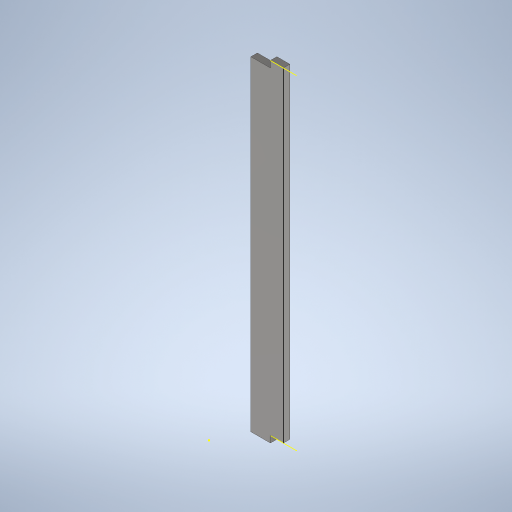
# Autodesk Inventor part: Part2
Saved by Autodesk Inventor 2024 (Build 280153000, 153)
## iProperties
Created: 2023-10-19
Part Number: Part2
Material: Steel, Carbon
Document SubType Name: Modeling
Designer: liuyu
Density: 7.85 g/cm^3
Appearance: Semi-Polished
Author: liuyu
Autodesk Inventor part; units mm, degrees
ref_plane "YZ Plane" through (0, 0, 0) normal (1, 0, 0) x (0, 1, 0)
ref_plane "XZ Plane" through (0, 0, 0) normal (0, 1, 0) x (-1, 0, 0)
ref_plane "XY Plane" through (0, 0, 0) normal (0, 0, 1) x (1, 0, 0)
sketch "Sketch1" plane through (0, 0, 0) normal (0, 0, 1) x (1, 0, 0)
  line L0 (32.1184, 271.7487) -> (82.1184, 271.7487)
  line L1 (82.1184, 271.7487) -> (82.1184, 21.7487)
  line L2 (82.1184, 21.7487) -> (32.1184, 21.7487)
  line L3 (32.1184, 21.7487) -> (32.1184, 271.7487)
  point P0 (0, 0)
  dimension "d0" = 50
  dimension "d1" = 250
  constraints: 8 end point, 2 parallel, 1 horizontal, 1 perpendicular
  measures "d0" distance of L1.end L2.end
  measures "d1" distance of L0.end L1.end
extrude "Extrusion1" add sketch "Sketch1" along normal blind 5
sketch "Sketch2" plane through (0, 0, 5) normal (0, 0, 1) x (1, 0, 0)
  line L0 (82.1184, 271.7487) -> (32.1184, 271.7487) projected
  line L1 (57.1184, 271.7487) -> (47.1184, 271.7487)
  line L2 (47.1184, 271.7487) -> (47.1184, 276.7487)
  line L3 (47.1184, 276.7487) -> (67.1184, 276.7487)
  line L4 (67.1184, 276.7487) -> (67.1184, 271.7487)
  line L5 (32.1184, 21.7487) -> (82.1184, 21.7487) projected
  line L6 (32.1184, 21.7487) -> (32.1184, 16.7487)
  line L7 (32.1184, 16.7487) -> (47.1184, 16.7487)
  line L8 (47.1184, 16.7487) -> (47.1184, 21.7487)
  line L9 (82.1184, 21.7487) -> (82.1184, 16.7487)
  line L10 (82.1184, 16.7487) -> (67.1184, 16.7487)
  line L11 (67.1184, 16.7487) -> (67.1184, 21.7487)
  point P0 (0, 0)
  dimension "d4" = 10
  dimension "d5" = 5
  dimension "d6" = 20
  dimension "d7" = 5
  dimension "d8" = 15
  dimension "d9" = 5
  dimension "d10" = 15
  constraints: 20 end point, 6 point on line, 5 perpendicular, 1 horizontal, 1 midpoint, 1 vertical
  measures "d4" distance of L1.start L1.end
  measures "d5" distance of L1.end L2.end
  measures "d6" distance of L2.end L3.end
  measures "d7" distance of L5.start L6.end
  measures "d8" distance of L6.end L7.end
  measures "d9" distance of L5.end L9.end
  measures "d10" distance of L9.end L10.end
extrude "Extrusion2" add sketch "Sketch2" against normal blind 5 contours L0 L2 L3 L4
sketch "Sketch3" plane through (0, 0, 5) normal (0, 0, 1) x (1, 0, 0)
  line L0 (32.1184, 21.7487) -> (82.1184, 21.7487) projected
  line L1 (32.1184, 21.7487) -> (32.1184, 16.7487)
  line L2 (32.1184, 16.7487) -> (47.1184, 16.7487)
  line L3 (47.1184, 16.7487) -> (47.1184, 21.7487)
  line L4 (82.1184, 21.7487) -> (82.1184, 16.7487)
  line L5 (82.1184, 16.7487) -> (67.1184, 16.7487)
  line L6 (67.1184, 16.7487) -> (67.1184, 21.7487)
  point P0 (0, 0)
  dimension "d13" = 5
  dimension "d14" = 15
  dimension "d15" = 5
  dimension "d16" = 15
  constraints: 12 end point, 4 perpendicular, 2 point on line, 2 vertical
  measures "d13" distance of L0.start L1.end
  measures "d14" distance of L1.end L2.end
  measures "d15" distance of L0.end L4.end
  measures "d16" distance of L4.end L5.end
extrude "Extrusion3" add sketch "Sketch3" against normal blind 5
sketch "Sketch4" plane through (0, 0, 5) normal (0, 0, 1) x (1, 0, 0)
  line L0 (47.1184, 21.7487) -> (67.1184, 21.7487) projected
  line L1 (57.1184, 21.7487) -> (57.1184, 26.7487)
  line L2 (57.1184, 26.7487) -> (47.1184, 26.7487)
  line L3 (47.1184, 26.7487) -> (47.1184, 21.7487)
  line L4 (47.1184, 21.7487) -> (67.1184, 21.7487)
  line L5 (67.1184, 21.7487) -> (67.1184, 26.7487)
  line L6 (67.1184, 26.7487) -> (57.1184, 26.7487)
  line L7 (47.1184, 21.7487) -> (32.1184, 21.7487)
  line L8 (32.1184, 21.7487) -> (82.1184, 21.7487)
  line L9 (82.1184, 16.7487) -> (82.1184, 271.7487) projected
  point P0 (0, 0)
  dimension "d19" = 5
  dimension "d20" = 10
  dimension "d21" = 15
  constraints: 16 end point, 4 point on line, 3 perpendicular, 1 collinear, 1 midpoint, 1 vertical
  measures "d19" distance of L1.start L1.end
  measures "d20" distance of L1.end L2.end
  measures "d21" distance of L0.start L7.end
sketch "Sketch5" plane through (0, 0, 5) normal (0, 0, 1) x (1, 0, 0)
  point P0 (0, 0)
sketch "Sketch6" plane through (0, 0, 5) normal (0, 0, 1) x (1, 0, 0)
  line L0 (47.1184, 21.7487) -> (67.1184, 21.7487) projected
  line L1 (47.1184, 21.7487) -> (47.1184, 16.7487) projected
  line L2 (47.1184, 21.7487) -> (47.1184, 16.7487)
  line L3 (32.1184, 271.7487) -> (32.1184, 16.7487) projected
  line L4 (47.1184, 16.7487) -> (32.1184, 16.7487)
  line L5 (32.1184, 16.7487) -> (32.1184, 21.7487)
  line L6 (47.1184, 21.7487) -> (32.1184, 21.7487)
  line L7 (32.1184, 21.7487) -> (32.1184, 16.7487)
  line L8 (32.1184, 16.7487) -> (47.1184, 16.7487)
  point P0 (0, 0)
  constraints: 12 end point, 4 perpendicular, 1 point on line, 1 vertical
extrude "Extrusion4" cut sketch "Sketch6" against normal blind 15
extrude "Extrusion5" cut sketch "Sketch4" against normal blind 15
sketch "Sketch7" plane through (0, 0, 5) normal (0, 0, 1) x (1, 0, 0)
  line L0 (67.1184, 26.7487) -> (67.1184, 16.7487) projected
  line L1 (67.1184, 21.7487) -> (67.1184, 16.7487)
  line L2 (82.1184, 16.7487) -> (82.1184, 271.7487) projected
  line L3 (67.1184, 16.7487) -> (82.1184, 16.7487)
  line L4 (82.1184, 16.7487) -> (82.1184, 21.7487)
  line L5 (67.1184, 21.7487) -> (82.1184, 21.7487)
  point P0 (0, 0)
  constraints: 8 end point, 2 perpendicular, 1 collinear, 1 midpoint, 1 point on line
extrude "Extrusion6" cut sketch "Sketch7" against normal blind 15
sketch "Sketch8" plane through (0, 0, 5) normal (0, 0, 1) x (1, 0, 0)
  line L0 (47.1184, 276.7487) -> (67.1184, 276.7487) projected
  line L1 (57.1184, 276.7487) -> (57.1184, 26.7487)
  line L2 (67.1184, 26.7487) -> (47.1184, 26.7487) projected
  point P0 (0, 0)
  constraints: 2 end point, 2 midpoint
sketch "Sketch9" plane through (0, 0, 5) normal (0, 0, 1) x (1, 0, 0)
  line L0 (47.1184, 276.7487) -> (67.1184, 276.7487) projected
  line L1 (57.1184, 276.7487) -> (57.1184, 26.7487)
  line L2 (67.1184, 26.7487) -> (47.1184, 26.7487) projected
  line L3 (67.1184, 21.7487) -> (67.1184, 26.7487) projected
  line L4 (67.1184, 26.7487) -> (67.1184, 21.7487)
  line L5 (82.1184, 271.7487) -> (82.1184, 21.7487) projected
  line L6 (67.1184, 21.7487) -> (82.1184, 21.7487)
  line L7 (82.1184, 21.7487) -> (82.1184, 271.7487)
  line L8 (82.1184, 271.7487) -> (67.1184, 271.7487)
  line L9 (67.1184, 271.7487) -> (67.1184, 276.7487)
  line L10 (67.1184, 276.7487) -> (57.1184, 276.7487)
  line L11 (67.1184, 276.7487) -> (67.1184, 271.7487)
  point P0 (0, 0)
  constraints: 16 end point, 5 perpendicular, 2 midpoint, 2 point on line, 1 vertical
extrude "Extrusion7" cut sketch "Sketch9" against normal blind 15
equation "\"d22\" = d21"
equation "\"d24\" = d21"
equation "\"d26\" = d21"
equation "\"d28\" = d21"
body "Solid1"
